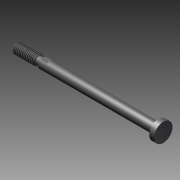
# Autodesk Inventor part: 16N2A12A010-(N0-pistone)
Saved by Autodesk Inventor 2011 SP1 (Build 150282100, 282)
## iProperties
Created: 2018-01-08
Part Number: 16N2A12A010-(N0-pistone)
Catalog Web Link: www.cadenas.de
Description: Minicylinders Serie 16 - 24 - 25 Single and double acting  Cetop RP52-P DIN/ISO 6432-Rod-
Vendor: CAMOZZI
Document SubType Name: Modeling
Designer: psAdmin
Manufacturer: CAMOZZI
Mass: 2.68664 g
Surface Area: 19.1906 cm^2
Volume: 2.68664 cm^3
Density: 1 g/cm^3
Category: PARTsolutions
Company: CAMOZZI
Title: 16N2A12A010
Author: Cadenas PARTsolutions
PSOL_IDENT_0: {$CADENAS_DATA\23d-libs\camozzi\movimento\cilindri_a_norma_e_cilindri_standard\minicilindri_serie_16
PSOL_IDENT_1: _24_25\minicilindr_serie_16_24_25_pistone.prj},283 {VTYP=3D},{NB=16N2A12A010-(N0-pistone)},{LINA=16N
PSOL_IDENT_2: 2A12A010},{NN=Minicylinders Serie 16 - 24 - 25 Single and double acting  Cetop RP52-P DIN/ISO 6432-R
PSOL_IDENT_3: od},{DATE=27.07.2017 08:45:31},{GEOMDATE=27.09.2013 11:24:00},{VERSION=},{LINEID=40},{LINESUBID=-1},
PSOL_IDENT_4: {WBVAR=FUNZ,HUBT,HUB,TYP,LSTELO}  {NB=16N2A12A010-(N0-pistone)},{LINA=16N2A12A010},{KT=DUMMY},{IDNR=
PSOL_IDENT_5: },{SERIE=16},{PHY=12},{EW=12},{KW=8},{BE=M16x1.5},{BENDM=16.000},{BEKDM=14.160},{KK=M6x1},{KKNDM=6.0
PSOL_IDENT_6: 00},{KKDM=4.773},{CD=6},{VERSION=N = standard},{FUNZ=2},{HUBT=N},{HUB=10},{MAT=A = stelo INOX rullat
PSOL_IDENT_7: o - camicia inox},{TYP=A},{V=V = guarnizione stelo viton},{D1=14.0},{EE=M5},{D3=6},{EENDM=5.000},{EE
PSOL_IDENT_8: KDM=4.019},{D2=6},{L1=105.0},{L11=105.0},{L12=126.0},{L13=0.000},{XC=75},{XC1=75},{XC2=0.000},{L2=50
PSOL_IDENT_9: .0},{AM=16},{L3=15},{L4=4.5},{L5=17},{L5X1=17},{L5X2=0.000},{L=9},{WF=22},{WF1=22},{WF2=0.000},{L6=9
PSOL_IDENT_10: },{L7=38},{L7X1=38},{L7X2=0.000},{KV=24},{SW=5},{SWIN=5.000},{D=20},{HUBA=-},{FIN=1,'1=semplice effe
PSOL_IDENT_11: tto',2,'2=doppio effetto',3,'3=doppio effetto stelo passante',7,'7=s.e. stelo passante'},{HUBIN=10,2
PSOL_IDENT_12: 5,40,50,80,100,125,160,200,250,300},{HUBIN1=10,25,40,50},{HUBIN2=[10:50]},{HUBIN3=10,25,40,50,80,100
PSOL_IDENT_13: ,125,160,200,250,300},{HUBIN4=[10:300]},{INFO=Infotext},{TYPIN1= 'A', 'A=ghiera V + dado stelo U'},{
PSOL_IDENT_14: TYPIN2= 'A', 'A=ghiera V + dado stelo U'},{TYPIN= 'A', 'A=ghiera V + dado stelo U'},{PRA=1},{HUBX=01
PSOL_IDENT_15: 0},{PHYX=12},{LSTELO=0},{LSTELOX=[0-1000]}
NN: Minicylinders Serie 16 - 24 - 25 Single and double acting  Cetop RP52-P DIN/ISO 6432-Rod
NB: 16N2A12A010-(N0-pistone)
NBSYN: $SERIE.N$FUNZ.A$PHYX.$TYP.$HUBX.-($HUBT.$LSTELO.-pistone)
LINA: 16N2A12A010
SERIE: 16
PHY: 12
EW: 12
KW: 8
BE: M16x1.5
KK: M6x1
CD: 6
VERSION: N = standard
FUNZ: 2=doppio effetto
HUBT: standard
HUB: 10
MAT: A = stelo INOX rullato - camicia inox
TYP: A=ghiera V + dado stelo U
V: V = guarnizione stelo viton
D1: 14.0
EE: M5
D3: 6
D2: 6
L1: 105.0
L13: 0.000
XC1: 75
XC2: 0.000
L2: 50.0
AM: 16
L3: 15
L4: 4.5
L5X1: 17
L5X2: 0.000
L: 9
WF1: 22
WF2: 0.000
L6: 9
L7X1: 38
L7X2: 0.000
KV: 24
SW: 5
SWIN: 5.000
D: 20
HUBA: -
INFO: Infotext
TYPIN1: 'A', 'A=ghiera V + dado stelo U'
TYPIN2: 'A', 'A=ghiera V + dado stelo U'
LSTELO: 0
SUPPLIER: CAMOZZI
ARTICLENO: 16N2A12A010-(N0-pistone)
BOMINFO: 16N2A12A010
CREATOR: CADENAS GmbH
Autodesk Inventor part; units mm, degrees
sketch "Skizze_1" plane through (0, 0, 0) normal (0, 0, 1) x (1, 0, 0)
  line L0 (51, 0) -> (-38, 0)
  line L1 (-38, 0) -> (-38, 2.3865)
  line L2 (-38, 2.3865) -> (-37.3865, 3)
  line L3 (-37.3865, 3) -> (-25.0135, 3)
  line L4 (-25.0135, 3) -> (-24.4, 2.3865)
  line L5 (-24.4, 2.3865) -> (-22, 2.3865)
  line L6 (-22, 2.3865) -> (-22, 3)
  line L7 (-22, 3) -> (48, 3)
  line L8 (48, 3) -> (48, 5.6)
  line L9 (48, 5.6) -> (51, 5.6)
  line L10 (51, 5.6) -> (51, 0)
  line L11 (51, 0) -> (-38, 0)
  constraints: 24 end point
revolve "Revolution1" add sketch "Skizze_1" angle 360 about axis through (51, 0, 0) along (1, 0, 0)
thread "Thread1" size "M6x1" class "6g" standard "ISO Metric profile" full length
sketch "Skizze_4" plane through (-22, 0, 0) normal (1, 0, 0) x (0, 0, -1)
  line L0 (-5, -16) -> (5, -16)
  line L1 (5, -16) -> (5, 16)
  line L2 (5, 16) -> (-5, 16)
  line L3 (-5, 16) -> (-5, -16)
  line L4 (-2.5, -8) -> (2.5, -8)
  line L5 (2.5, -8) -> (2.5, 8)
  line L6 (2.5, 8) -> (-2.5, 8)
  line L7 (-2.5, 8) -> (-2.5, -8)
  constraints: 16 end point
extrude "Extrusion1" cut sketch "Skizze_4" along normal blind 4
ref_plane "P1_XY" through (0, 0, 0) normal (1, 0, 0) x (0, 0, -1)
ref_plane "P1_YZ" through (0, 0, 0) normal (0, 0, -1) x (0, 1, 0)
ref_plane "P1_ZX" through (0, 0, 0) normal (0, 1, 0) x (1, 0, 0)
ref_plane "PD1_XY" through (-32, 0, 0) normal (1, 0, 0) x (0, 0, -1)
ref_plane "PD1_YZ" through (-32, 0, 0) normal (0, 0, -1) x (0, 1, 0)
ref_plane "PD1_ZX" through (-32, 0, 0) normal (0, 1, 0) x (1, 0, 0)
ref_plane "PD2_XY" through (102, 0, 0) normal (1, 0, 0) x (0, 0, -1)
ref_plane "PD2_YZ" through (102, 0, 0) normal (0, 0, -1) x (0, 1, 0)
ref_plane "PD2_ZX" through (102, 0, 0) normal (0, 1, 0) x (1, 0, 0)
body "Solid1"
